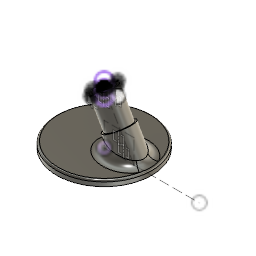
base-plate (Autodesk Fusion 360 design; units mm, degrees)
Autodesk Fusion 360 part; units mm, degrees
sketch "Skizze1" plane through (0, 0, 0) normal (0, 0, 1) x (1, 0, 0)
  circle A0 centre (0, 0) radius 80
  dimension "d1" = 160
  constraint coincident A0.centre origin
  measures "d1" diameter of A0
extrude "Extrusion1" add sketch "Skizze1" along normal blind 10
fillet "Abrundung1" radius 3 1 edges at (-74.5862, -28.9292, 10)
sketch "Skizze2" plane through (0, 0, 0) normal (0, 1, 0) x (1, 0, 0)
  line L0 (0, 0) -> (50, 0) construction
  line L1 (50, 0) -> (50, -40) construction
  line L2 (50, -40) -> (0, -40) construction
  line L3 (0, -40) -> (0, 0) construction
  line L4 (50, 0) -> (0, -86.6025) construction
  line L5 (50, 0) -> (160, 0) construction
  line L6 (0, -86.6025) -> (19.9186, -98.1025)
  line L7 (0, -86.6025) -> (23, -86.6025) construction
  line L8 (0, -86.6025) -> (-19.9186, -75.1025)
  dimension "d6" = 50
  dimension "d7" = 40
  dimension "d8" = 120
  dimension "d9" = 100
  dimension "d10" = 30
  dimension "d11" = 23
  constraint horizontal L0
  constraint vertical L1
  constraint horizontal L2
  constraint vertical L3
  constraint coincident L0.start L3.end
  constraint horizontal L5
  constraint horizontal L7
  constraint symmetric L6.start L4 L7.start
  constraint symmetric L4 L6.end L8.end
  measures "d6" distance of L0.start L0.end
  measures "d7" distance of L0.start L2.end
  measures "d8" angle of L4 L5
  measures "d9" distance of L0.end L4.end
  measures "d10" angle of L6 L7
  measures "d11" distance of L4.end L6.end
sketch "Skizze3" plane through (0, 0, 0) normal (1, 0, 0) x (0, 1, 0)
  line L0 (0, 86.6025) -> (0, 75.1025)
  line L1 (0, 86.6025) -> (0, 98.1025)
  line L2 (0, 86.6025) -> (-23, 86.6025)
  line L3 (0, 86.6025) -> (23, 86.6025)
  point P0 (0, 75.1025)
  point P1 (0, 86.6025)
  dimension "d12" = 23
  dimension "d13" = 23
  constraint coincident P1 L0.start
  constraint perpendicular L0 L2
  constraint perpendicular L0 L3
  measures "d12" distance of P1 L2.end
  measures "d13" distance of P1 L3.end
ref_plane "Arbeitsebene1" through (0, 0, 86.6025) normal (0.5, 0, -0.866025) x (0, 1, 0)
sketch "Skizze4" plane through (-37.5, 0, 64.9519) normal (0.5, 0, -0.866025) x (0, 1, 0)
  line L0 (0, 43.3013) -> (23, 43.3013)
  line L1 (0, 43.3013) -> (-23, 43.3013)
  line L2 (0, 43.3013) -> (0, 20.3013)
  line L3 (0, 43.3013) -> (0, 66.3013)
  circle A0 centre (0, 43.3013) radius 23
  circle A1 centre (0, 43.3013) radius 15.75
  circle A2 centre (0, 43.3013) radius 20
  point P0 (23, 43.3013)
  point P1 (0, 20.3013)
  point P2 (-23, 43.3013)
  point P3 (0, 66.3013)
  point P4 (0, 43.3013)
  dimension "d15" = 46
  dimension "d20" = 31.5
  dimension "d21" = 40
  constraint coincident P4 L0.start
  measures "d15" diameter of A0
  measures "d20" diameter of A1
  measures "d21" diameter of A2
extrude "Extrusion2" add sketch "Skizze4" along normal blind 120
fillet "Abrundung2" radius 15 1 edges at (17.6684, 0, 10)
sketch "Skizze5" plane through (-37.5, 0, 64.9519) normal (-0.5, 0, 0.866025) x (0, -1, 0)
  circle A0 centre (0, 43.3013) radius 23
  circle A1 centre (0, 43.3013) radius 15.75
  dimension "d22" = 31.5
  constraint concentric A0 A1
  measures "d22" diameter of A1
extrude "Extrusion3" cut sketch "Skizze5" against normal blind 170 contours A1
sketch "Skizze6" plane through (-37.5, 0, 64.9519) normal (-0.5, 0, 0.866025) x (0, -1, 0)
  circle A0 centre (0, 43.3013) radius 15.75
  circle A1 centre (0, 43.3013) radius 23
  circle A2 centre (0, 43.3013) radius 20
  dimension "d25" = 40
  constraint concentric A0 A2
  measures "d25" diameter of A2
extrude "Extrusion4" cut sketch "Skizze6" against normal blind 50 contours A1
sketch "Skizze7" plane through (0, 0, 0) normal (0, 0, 1) x (1, 0, 0)
  line L0 (-80, 80) -> (111.2852, 80)
  line L1 (111.2852, 80) -> (111.2852, -85.555)
  line L2 (111.2852, -85.555) -> (-80, -85.555)
  line L3 (-80, -85.555) -> (-80, 80)
  constraint horizontal L0
  constraint vertical L1
  constraint horizontal L2
  constraint vertical L3
extrude "Extrusion5" cut sketch "Skizze7" against normal blind 90
